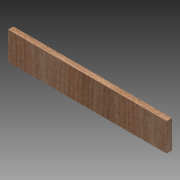
# Autodesk Inventor part: Robot-Base-BatteryBack
Saved by Autodesk Inventor 2012 (Build 160160000, 160)
## iProperties
Created: 2013-07-14
Part Number: Robot-Base-BatteryBack
Material: Wood (Birch)
Document SubType Name: Modeling
Designer: joe_000
Density: 0.55 g/cm^3
Mass: 179.87 g
Surface Area: 628.958 cm^2
Volume: 327.036 cm^3
Author: joe_000
Autodesk Inventor part; units mm, degrees
ref_plane "YZ Plane" through (0, 0, 0) normal (1, 0, 0) x (0, 1, 0)
ref_plane "XZ Plane" through (0, 0, 0) normal (0, 1, 0) x (-1, 0, 0)
ref_plane "XY Plane" through (0, 0, 0) normal (0, 0, 1) x (1, 0, 0)
sketch "Sketch1" plane through (0, 0, 0) normal (1, 0, 0) x (0, 1, 0)
  line L0 (0, 0) -> (67.5875, 0)
  line L1 (67.5875, 0) -> (67.5875, -12.7)
  line L2 (67.5875, -12.7) -> (0, -12.7)
  line L3 (0, -12.7) -> (0, 0)
  dimension "d0" = 12.7
  dimension "d1" = 67.5875
  constraints: 8 end point, 2 parallel, 1 horizontal, 1 perpendicular
  measures "d0" distance of L0.end L1.end
  measures "d1" distance of L1.end L2.end
extrude "Extrusion1" add sketch "Sketch1" along normal blind 381
equation "\"d0\" = BaseSupportThickness"
equation "\"d1\" = BaseSupportHeight"
equation "\"d2\" = BaseWidth - 2 * BaseSupportThickness"
equation "\"BaseSupportThickness\" = 12.7"
equation "\"BaseSupportHeight\" = 67.5875"
equation "\"BaseWidth\" = 406.4"
body "Solid1"
